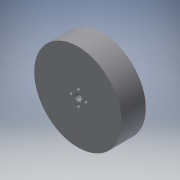
# Autodesk Inventor part: AM Wheel
Saved by Autodesk Inventor 2016 (Build 200138000, 138)
## iProperties
Created: 2016-01-08
Part Number: AM Wheel
Material: Generic
Document SubType Name: Modeling
Designer: TimB
Density: 1 g/cm^3
Appearance: Default
Author: TimB
Autodesk Inventor part; units mm, degrees
ref_plane "YZ Plane" through (0, 0, 0) normal (1, 0, 0) x (0, 1, 0)
ref_plane "XZ Plane" through (0, 0, 0) normal (0, 1, 0) x (-1, 0, 0)
ref_plane "XY Plane" through (0, 0, 0) normal (0, 0, 1) x (1, 0, 0)
sketch "Sketch1" plane through (0, 0, 0) normal (0, 1, 0) x (-1, 0, 0)
  circle A0 centre (0, 0) radius 47
  circle A1 centre (0, 0) radius 4 projected
  circle A2 centre (0, 8) radius 1.85 projected
  circle A3 centre (-8, 0) radius 1.85 projected
  circle A4 centre (8, 0) radius 1.85 projected
  circle A5 centre (0, -8) radius 1.85 projected
  dimension "d0" = 94
  constraints: 1 centre point, 1 coincident
  measures "d0" diameter of A0
extrude "Extrusion2" add sketch "Sketch1" along normal blind 26
body "Solid2"
